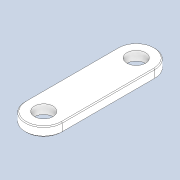
# Autodesk Inventor part: LINK
Saved by Autodesk Inventor 2021 (Build 250183000, 183)
## iProperties
Created: 2020-05-02
Part Number: LINK
Material: Aluminium 6082 T6
Document SubType Name: Modeling
Designer: Hannah
Density: 2.7 g/cm^3
Appearance: Aluminum - Dark
Mass: 15.5114 g
Surface Area: 33.4644 cm^2
Volume: 5.74495 cm^3
Vendor: Custom
Description: seatpost clamp link
Author: Hannah
Revision Number: 1
Autodesk Inventor part; units mm, degrees
ref_plane "YZ Plane" through (0, 0, 0) normal (1, 0, 0) x (0, 1, 0)
ref_plane "XZ Plane" through (0, 0, 0) normal (0, 1, 0) x (-1, 0, 0)
ref_plane "XY Plane" through (0, 0, 0) normal (0, 0, 1) x (1, 0, 0)
sketch "Sketch1" plane through (0, 0, 0) normal (0, 1, 0) x (-1, 0, 0)
  circle A0 centre (0, 25) radius 5
  arc A1 (10, 25) -> (-10, 25) centre (0, 25) ccw
  arc A2 (-10, -25) -> (10, -25) centre (0, -25) ccw
  circle A3 centre (0, -25) radius 5
  line L0 (10, 25) -> (10, -25)
  line L1 (-10, -25) -> (-10, 25)
  line L2 (10, 25) -> (10, 35)
  line L3 (-10, 25) -> (-10, 35)
  line L4 (-10, 35) -> (10, 35)
  line L5 (-10, -25) -> (-10, -35)
  line L6 (-10, -35) -> (10, -35)
  line L7 (10, -35) -> (10, -25)
  point P0 (0, 0)
  point P1 (10, 0)
  point P2 (0, -35)
  point P3 (0, 35)
  dimension "d0" = 50
  dimension "d1" = 10
  dimension "d2" = 20
  constraints: 16 end point, 7 point on circle, 5 tangent, 4 centre point, 4 point on line, 4 vertical, 3 perpendicular, 2 coincident, 2 equal radius, 2 vertical alignment, 1 horizontal alignment, 1 midpoint
  measures "d0" distance of A2.centre A0.centre
  measures "d1" diameter of A0
  measures "d2" diameter of A1
extrude "Extrusion1" add sketch "Sketch1" along normal mid plane 5 contours L0 A2 L1 A1
extrude "Extrusion2" [suppressed]
chamfer "Chamfer1" distance 0.5 angle 45 8 edges at (-10, -2.5, 0) (0, -2.5, -35) (0, -2.5, 35) (10, -2.5, 0) (-10, 2.5, 0) (0, 2.5, 35) (10, 2.5, 0) (0, 2.5, -35)
body "Solid1"
